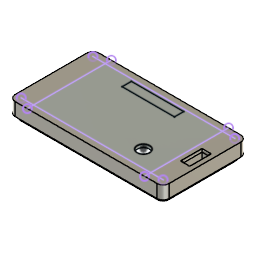
Flashlight (Autodesk Fusion 360 design; units mm, degrees)
Autodesk Fusion 360 part; units mm, degrees
note: some values were not read from the file. Set by a fixed rule: which sketch regions a step uses.
sketch "Sketch1" plane through (0, 0, 0) normal (0, 0, 1) x (1, 0, 0) in component "Bottom"
  line L0 (0, 0) -> (38.1, 0)
  line L1 (38.1, 0) -> (38.1, 27.3)
  line L2 (38.1, 27.3) -> (0, 27.3)
  line L3 (0, 27.3) -> (0, 0)
  line L4 (0, 0) -> (-4, 0)
  line L5 (-6, 2) -> (-6, 25.3)
  line L6 (-4, 27.3) -> (0, 27.3)
  line L7 (0, 27.3) -> (0, 0)
  line L8 (38.1, 0) -> (42.1, 0)
  line L9 (44.1, 2) -> (44.1, 25.3)
  line L10 (42.1, 27.3) -> (38.1, 27.3)
  line L11 (38.1, 27.3) -> (38.1, 0)
  line L12 (-4, 2) -> (42.1, 2)
  line L13 (42.1, 2) -> (42.1, 25.3)
  line L14 (42.1, 25.3) -> (-4, 25.3)
  line L15 (-4, 25.3) -> (-4, 2)
  line L16 (-4, 2) -> (0, 2)
  line L17 (0, 2) -> (0, 5)
  line L18 (-1, 6) -> (-4, 6)
  line L19 (-4, 6) -> (-4, 2)
  line L20 (-4, 25.3) -> (0, 25.3)
  line L21 (0, 25.3) -> (0, 22.3)
  line L22 (-1, 21.3) -> (-4, 21.3)
  line L23 (-4, 21.3) -> (-4, 25.3)
  line L24 (42.1, 25.3) -> (38.1, 25.3)
  line L25 (38.1, 25.3) -> (38.1, 22.3)
  line L26 (39.1, 21.3) -> (42.1, 21.3)
  line L27 (42.1, 21.3) -> (42.1, 25.3)
  line L28 (42.1, 2) -> (38.1, 2)
  line L29 (38.1, 2) -> (38.1, 5)
  line L30 (39.1, 6) -> (42.1, 6)
  line L31 (42.1, 6) -> (42.1, 2)
  arc A0 (-1, 21.3) -> (0, 22.3) centre (-1, 22.3) ccw
  arc A1 (38.1, 22.3) -> (39.1, 21.3) centre (39.1, 22.3) ccw
  arc A2 (39.1, 6) -> (38.1, 5) centre (39.1, 5) ccw
  arc A3 (0, 5) -> (-1, 6) centre (-1, 5) ccw
  arc A4 (-4, 27.3) -> (-6, 25.3) centre (-4, 25.3) ccw
  arc A5 (44.1, 25.3) -> (42.1, 27.3) centre (42.1, 25.3) ccw
  arc A6 (42.1, 0) -> (44.1, 2) centre (42.1, 2) ccw
  arc A7 (-6, 2) -> (-4, 0) centre (-4, 2) ccw
  line L32 (-3.5, 26.55) -> (41.6, 26.55)
  line L33 (43.35, 24.8) -> (43.35, 2.5)
  line L34 (41.6, 0.75) -> (-3.5, 0.75)
  line L35 (-5.25, 2.5) -> (-5.25, 24.8)
  arc A8 (-3.5, 26.55) -> (-5.25, 24.8) centre (-3.5, 24.8) ccw
  arc A9 (43.35, 24.8) -> (41.6, 26.55) centre (41.6, 24.8) ccw
  arc A10 (41.6, 0.75) -> (43.35, 2.5) centre (41.6, 2.5) ccw
  arc A11 (-5.25, 2.5) -> (-3.5, 0.75) centre (-3.5, 2.5) ccw
  line L36 (-1, 19) -> (22, 19)
  line L37 (22, 19) -> (22, 6.5)
  line L38 (22, 6.5) -> (-1, 6.5)
  line L39 (-1, 6.5) -> (-1, 19)
  line L40 (-1, 19) -> (22, 19)
  line L41 (22, 19) -> (22, 19.5)
  line L42 (22, 19.5) -> (-1, 19.5)
  line L43 (-1, 19.5) -> (-1, 19)
  line L44 (-1, 6.5) -> (22, 6.5)
  line L45 (22, 6.5) -> (22, 6)
  line L46 (22, 6) -> (-1, 6)
  line L47 (-1, 6) -> (-1, 6.5)
  line L48 (22, 19) -> (21.5, 19)
  line L49 (21.5, 19) -> (21.5, 6.5)
  line L50 (21.5, 6.5) -> (22, 6.5)
  line L51 (22, 6.5) -> (22, 19)
  line L52 (38.1, 25.3) -> (28.1, 25.3)
  line L53 (28.1, 25.3) -> (28.1, 23.3)
  line L54 (28.1, 23.3) -> (38.1, 23.3)
  line L55 (38.1, 23.3) -> (38.1, 25.3)
  line L56 (38.1, 2) -> (28.1, 2)
  line L57 (28.1, 2) -> (28.1, 4)
  line L58 (28.1, 4) -> (38.1, 4)
  line L59 (38.1, 4) -> (38.1, 2)
  line L60 (42.1, 18.65) -> (38.1, 18.65)
  line L61 (38.1, 18.65) -> (38.1, 8.65)
  line L62 (38.1, 8.65) -> (42.1, 8.65)
  line L63 (42.1, 8.65) -> (42.1, 18.65)
  line L64 (42.1, 16.65) -> (40.1, 16.65)
  line L65 (40.1, 16.65) -> (40.1, 10.65)
  line L66 (40.1, 10.65) -> (42.1, 10.65)
  line L67 (42.1, 10.65) -> (42.1, 16.65)
  point P0 (-6, 0)
  point P1 (-6, 27.3)
  point P2 (44.1, 0)
  point P3 (44.1, 27.3)
  point P4 (-5.25, 26.55)
  point P5 (43.35, 26.55)
  point P6 (-5.25, 0.75)
  dimension "d1" = 38.1
  dimension "d2" = 27.3
  dimension "d3" = 6
  dimension "d4" = 27.3
  dimension "d5" = 6
  dimension "d6" = 27.3
  dimension "d8" = 46.1
  dimension "d9" = 23.3
  dimension "d10" = 50.1
  dimension "d11" = 2
  dimension "d12" = 2
  dimension "d13" = 4
  dimension "d14" = 4
  dimension "d15" = 4
  dimension "d16" = 4
  dimension "d17" = 4
  dimension "d18" = 4
  dimension "d19" = 4
  dimension "d20" = 4
  dimension "d21" = 1
  dimension "d22" = 1
  dimension "d23" = 1
  dimension "d24" = 1
  dimension "d25" = 2
  dimension "d26" = 2
  dimension "d27" = 2
  dimension "d28" = 2
  dimension "d29" = 48.6
  dimension "d30" = 25.8
  dimension "d31" = 0.75
  dimension "d32" = 0.75
  dimension "d33" = 1.75
  dimension "d34" = 1.75
  dimension "d35" = 1.75
  dimension "d36" = 1.75
  dimension "d37" = 23
  dimension "d38" = 12.5
  dimension "d39" = 4.5
  dimension "d40" = 3
  dimension "d41" = 23
  dimension "d42" = 0.5
  dimension "d43" = 23
  dimension "d44" = 0.5
  dimension "d45" = 0.5
  dimension "d46" = 12.5
  dimension "d47" = 10
  dimension "d48" = 2
  dimension "d49" = 10
  dimension "d50" = 2
  dimension "d90" = 15.3
  dimension "d91" = 4
  dimension "d92" = 10
  dimension "d93" = 2.65
  dimension "d94" = 2
  dimension "d95" = 6
  dimension "d96" = 2
  constraint horizontal L0
  constraint vertical L1
  constraint horizontal L2
  constraint vertical L3
  constraint coincident L0.start L3.end
  constraint horizontal L4
  constraint vertical L5
  constraint horizontal L6
  constraint vertical L7
  constraint horizontal L8
  constraint vertical L9
  constraint horizontal L10
  constraint vertical L11
  constraint horizontal L12
  constraint vertical L13
  constraint horizontal L14
  constraint vertical L15
  constraint horizontal L16
  constraint vertical L17
  constraint horizontal L18
  constraint vertical L19
  constraint horizontal L20
  constraint vertical L21
  constraint horizontal L22
  constraint vertical L23
  constraint horizontal L24
  constraint vertical L25
  constraint horizontal L26
  constraint vertical L27
  constraint horizontal L28
  constraint vertical L29
  constraint horizontal L30
  constraint vertical L31
  constraint tangent L21 A0
  constraint tangent L22 A0
  constraint tangent L25 A1
  constraint tangent L26 A1
  constraint tangent L29 A2
  constraint tangent L30 A2
  constraint tangent L17 A3
  constraint tangent L18 A3
  constraint coincident P1 L5
  constraint coincident P1 L6
  constraint tangent L5 A4
  constraint tangent L6 A4
  constraint coincident P3 L9
  constraint coincident P3 L10
  constraint tangent L9 A5
  constraint tangent L10 A5
  constraint coincident P2 L8
  constraint coincident P2 L9
  constraint tangent L8 A6
  constraint tangent L9 A6
  constraint coincident P0 L4
  constraint coincident P0 L5
  constraint tangent L4 A7
  constraint tangent L5 A7
  constraint horizontal L32
  constraint vertical L33
  constraint horizontal L34
  constraint vertical L35
  constraint coincident P4 L32
  constraint coincident P4 L35
  constraint tangent L32 A8
  constraint tangent L35 A8
  constraint coincident P5 L32
  constraint coincident P5 L33
  constraint tangent L32 A9
  constraint tangent L33 A9
  constraint tangent L33 A10
  constraint tangent L34 A10
  constraint coincident P6 L34
  constraint coincident P6 L35
  constraint tangent L34 A11
  constraint tangent L35 A11
  constraint horizontal L36
  constraint vertical L37
  constraint horizontal L38
  constraint vertical L39
  constraint horizontal L40
  constraint vertical L41
  constraint horizontal L42
  constraint vertical L43
  constraint horizontal L44
  constraint vertical L45
  constraint horizontal L46
  constraint vertical L47
  constraint horizontal L48
  constraint vertical L49
  constraint horizontal L50
  constraint vertical L51
  constraint horizontal L52
  constraint vertical L53
  constraint horizontal L54
  constraint vertical L55
  constraint horizontal L56
  constraint vertical L57
  constraint horizontal L58
  constraint vertical L59
  constraint horizontal L60
  constraint vertical L61
  constraint horizontal L62
  constraint vertical L63
  constraint coincident L13 L60.start
  constraint horizontal L64
  constraint vertical L65
  constraint horizontal L66
  constraint vertical L67
  constraint coincident L63 L64.start
  measures "d1" distance of L0.start L0.end
  measures "d2" distance of L0.start L2.end
  measures "d3" distance of L0.start P0
  measures "d4" distance of L0.start L2.end
  measures "d5" distance of L0.end P2
  measures "d6" distance of L0.end L1.end
  measures "d8" distance of L12.start L12.end
  measures "d9" distance of L12.start L14.end
  measures "d10" distance of P1 P3
  measures "d11" distance of L4 L12
  measures "d12" distance of L5 L15
  measures "d13" distance of L12.start L16.end
  measures "d14" distance of L12.start L18.end
  measures "d15" distance of L14.end L20.end
  measures "d16" distance of L14.end L22.end
  measures "d17" distance of L13.end L24.end
  measures "d18" distance of L13.end L26.end
  measures "d19" distance of L12.end L28.end
  measures "d20" distance of L12.end L30.end
  measures "d21" radius of A0
  measures "d22" radius of A1
  measures "d23" radius of A2
  measures "d24" radius of A3
  measures "d25" radius of A4
  measures "d26" radius of A5
  measures "d27" radius of A6
  measures "d28" radius of A7
  measures "d29" distance of P4 P5
  measures "d30" distance of P4 P6
  measures "d31" distance of L2 L32
  measures "d32" distance of L5 L35
  measures "d33" radius of A8
  measures "d34" radius of A9
  measures "d35" radius of A10
  measures "d36" radius of A11
  measures "d37" distance of L36.start L36.end
  measures "d38" distance of L36.start L38.end
  measures "d39" distance of L12 L38
  measures "d40" distance of L15 L39
  measures "d41" distance of L36.start L36.end
  measures "d42" distance of L36.start L42.end
  measures "d43" distance of L38.end L37.end
  measures "d44" distance of L38.end L18.start
  measures "d45" distance of L36.end L48.end
  measures "d46" distance of L36.end L37.end
  measures "d47" distance of L24.end L52.end
  measures "d48" distance of L24.end L54.end
  measures "d49" distance of L28.end L56.end
  measures "d50" distance of L28.end L58.end
  measures "d90" distance of L26 L30
  measures "d91" distance of L60.start L60.end
  measures "d92" distance of L60.start L62.end
  measures "d93" distance of L26 L60
  measures "d94" distance of L64.start L64.end
  measures "d95" distance of L64.start L66.end
  measures "d96" distance of L60 L64
extrude "Extrude1" add sketch "Sketch1" against normal blind 1 makes body 1 in component "Bottom"
extrude "Extrude2" add sketch "Sketch1" along normal blind 5.5 contours L3 L7 L38 L44 L46 L47 | L3 L7 L38 L44 L45 L46 L50 | L3 L7 L36 L40 L42 L43 | L3 L7 L36 L40 L41 L42 L48 | L36 L37 L38 L40 L44 L48 L49 L50 L51 bodies 1 in component "Bottom"
extrude "Extrude3" add sketch "Sketch1" along normal blind 5.5 contours L1 L11 L12 L29 L56 L57 L58 L59 | L1 L11 L14 L25 L52 L53 L54 L55 bodies 1 in component "Bottom"
extrude "Extrude4" add sketch "Sketch1" along normal blind 7.1 separate body contours L3 L7 L12 L14 L15 L16 L19 L20 L23 L32 L34 L35 A8 A11 | L1 L3 L7 L11 L12 L34 L56 | L1 L11 L12 L13 L14 L24 L27 L28 L31 L32 L33 L34 A9 A10 L63 L67 | L3 L7 L12 L15 L16 L17 L18 L19 A3 | L1 L11 L12 L13 L28 L29 L30 L31 A2 L59 | L3 L7 L14 L15 L20 L21 L22 L23 A0 | L1 L3 L7 L11 L14 L32 L52 | L1 L11 L13 L14 L24 L25 L26 L27 A1 L55 makes body 2 in component "Bottom"
extrude "Extrude5" add sketch "Sketch1" along normal blind 8.1 contours L0 L1 L3 L7 L11 L34 | L3 L4 L5 L6 L7 A4 A7 L32 L34 L35 A8 A11 | L1 L8 L9 L10 L11 A5 A6 L32 L33 L34 A9 A10 | L1 L2 L3 L7 L11 L32 bodies 1 2 in component "Bottom"
sketch "Sketch2" plane through (0, 0, 8.1) normal (0, 0, 1) x (-1, 0, 0) in component "Bottom"
  arc A0 (3.5, -26.55) -> (5.25, -24.8) centre (3.5, -24.8) ccw
  line L0 (3.5, -26.55) -> (-41.6, -26.55)
  arc A1 (-43.35, -24.8) -> (-41.6, -26.55) centre (-41.6, -24.8) ccw
  line L1 (-43.35, -24.8) -> (-43.35, -2.5)
  arc A2 (-41.6, -0.75) -> (-43.35, -2.5) centre (-41.6, -2.5) ccw
  line L2 (-41.6, -0.75) -> (3.5, -0.75)
  arc A3 (5.25, -2.5) -> (3.5, -0.75) centre (3.5, -2.5) ccw
  line L3 (5.25, -2.5) -> (5.25, -24.8)
  arc A4 (4, -27.3) -> (6, -25.3) centre (4, -25.3) ccw
  line L4 (6, -25.3) -> (6, -2)
  arc A5 (6, -2) -> (4, 0) centre (4, -2) ccw
  line L5 (4, 0) -> (-42.1, 0)
  arc A6 (-42.1, 0) -> (-44.1, -2) centre (-42.1, -2) ccw
  line L6 (-44.1, -2) -> (-44.1, -25.3)
  arc A7 (-44.1, -25.3) -> (-42.1, -27.3) centre (-42.1, -25.3) ccw
  line L7 (-42.1, -27.3) -> (4, -27.3)
  line L8 (-1, -27.3) -> (-9.2, -27.3)
  line L9 (-9.2, -27.3) -> (-9.2, -25.3)
  line L10 (-9.2, -25.3) -> (-1, -25.3)
  line L11 (-1, -25.3) -> (-1, -27.3)
  line L12 (0, -27.3) -> (0, 0)
  dimension "d61" = 8.2
  dimension "d62" = 2
  dimension "d63" = 1
  constraint horizontal L8
  constraint vertical L9
  constraint horizontal L10
  constraint vertical L11
  constraint coincident L7 L8.start
  measures "d61" distance of L8.start L8.end
  measures "d62" distance of L8.start L10.end
  measures "d63" distance of L11 L12
extrude "Extrude6" cut sketch "Sketch2" against normal blind 1.2 contours L0 L7 L8 L9 L11 | L0 L9 L10 L11 bodies 1 in component "Bottom"
sketch "Sketch3" plane through (0, 0, -1) normal (0, 0, -1) x (1, 0, 0) in component "Bottom"
  arc A0 (-6, -25.3) -> (-4, -27.3) centre (-4, -25.3) ccw
  line L0 (-4, -27.3) -> (42.1, -27.3)
  arc A1 (42.1, -27.3) -> (44.1, -25.3) centre (42.1, -25.3) ccw
  line L1 (44.1, -25.3) -> (44.1, -2)
  arc A2 (44.1, -2) -> (42.1, 0) centre (42.1, -2) ccw
  line L2 (42.1, 0) -> (-4, 0)
  arc A3 (-4, 0) -> (-6, -2) centre (-4, -2) ccw
  line L3 (-6, -2) -> (-6, -25.3)
  circle A4 centre (-3, -3) radius 2.5
  line L4 (0, 0) -> (-4, 0)
  line L5 (-6, -2) -> (-6, -25.3)
  circle A5 centre (-3, -3) radius 1
  circle A6 centre (41.1, -3) radius 2.5
  line L6 (38.1, 0) -> (42.1, 0)
  line L7 (44.1, -2) -> (44.1, -25.3)
  circle A7 centre (41.1, -3) radius 1
  circle A8 centre (41.1, -24.3) radius 2.5
  line L8 (42.1, -27.3) -> (38.1, -27.3)
  circle A9 centre (41.1, -24.3) radius 1
  circle A10 centre (-3, -24.3) radius 2.5
  line L9 (-4, -27.3) -> (0, -27.3)
  circle A11 centre (-3, -24.3) radius 1
  dimension "d66" = 5
  dimension "d67" = 3
  dimension "d68" = 3
  dimension "d69" = 2
  dimension "d70" = 5
  dimension "d71" = 3
  dimension "d72" = 3
  dimension "d73" = 2
  dimension "d74" = 5
  dimension "d75" = 3
  dimension "d76" = 3
  dimension "d77" = 2
  dimension "d78" = 5
  dimension "d79" = 3
  dimension "d80" = 3
  dimension "d81" = 2
  constraint concentric A4 A5
  constraint concentric A6 A7
  constraint concentric A8 A9
  constraint concentric A10 A11
  measures "d66" diameter of A4
  measures "d67" distance of A4.centre L4
  measures "d68" distance of A4.centre L5
  measures "d69" diameter of A5
  measures "d70" diameter of A6
  measures "d71" distance of A6.centre L6
  measures "d72" distance of A6.centre L7
  measures "d73" diameter of A7
  measures "d74" diameter of A8
  measures "d75" distance of L7 A8.centre
  measures "d76" distance of A8.centre L8
  measures "d77" diameter of A9
  measures "d78" diameter of A10
  measures "d79" distance of L5 A10.centre
  measures "d80" distance of A10.centre L9
  measures "d81" diameter of A11
extrude "Extrude7" cut sketch "Sketch3" against normal blind 9.5 contours A5 | A7 | A9 | A11 bodies 1 in component "Bottom"
extrude "Extrude8" cut sketch "Sketch3" against normal blind 5 contours A4 | A6 | A8 | A10 bodies 1 in component "Bottom"
chamfer "Chamfer1" distance 1.5 angle 45 1 edges at (-3.9323, 24.6616, 4) on bodies 1 in component "Bottom"
chamfer "Chamfer2" distance 1.5 angle 45 1 edges at (-3.9323, 3.3616, 4) on bodies 1 in component "Bottom"
chamfer "Chamfer3" distance 1.5 angle 45 1 edges at (40.1677, 24.6616, 4) on bodies 1 in component "Bottom"
chamfer "Chamfer4" distance 1.5 angle 45 1 edges at (40.1677, 3.3616, 4) on bodies 1 in component "Bottom"
extrude "Extrude9" cut sketch "Sketch1" against normal blind 1 contours L13 L63 L64 L65 L66 L67 bodies 1 in component "Bottom"
extrude "Extrude10" add sketch "Sketch1" along normal blind 7.1 separate body contours L1 L11 L13 L60 L61 L62 L63 L64 L65 L66 makes body 3 in component "Bottom"
fillet "Fillet1" radius 0.5 4 edges at (40.1, 13.65, -1) (41.1, 16.65, -1) (42.1, 13.65, -1) (41.1, 10.65, -1) on bodies 1 in component "Bottom"
sketch "Sketch1 (2)" plane through (0, 0, 0) normal (0, 0, 1) x (1, 0, 0) in component "Top"
  line L0 (-4, 6) -> (19, 6)
  arc A0 (-7, 26.8) -> (-9, 24.8) centre (-7, 24.8) ccw
  line L1 (39.1, 20.8) -> (39.1, 24.8)
  line L2 (39.1, 16.15) -> (37.1, 16.15)
  line L3 (39.1, 26.8) -> (35.1, 26.8)
  arc A1 (-6.25, 25.8) -> (-8, 24.05) centre (-6.25, 24.05) ccw
  line L4 (19, 6) -> (19, 5.5)
  line L5 (19, 18.5) -> (19, 6)
  line L6 (-7, 26.8) -> (-3, 26.8)
  arc A2 (-4, 20.8) -> (-3, 21.8) centre (-4, 21.8) ccw
  line L7 (39.1, 24.8) -> (-7, 24.8)
  line L8 (-9, 1.5) -> (-9, 24.8)
  line L9 (-3, 26.8) -> (-3, -0.5)
  arc A3 (38.35, 0.5) -> (40.1, 2.25) centre (38.35, 2.25) ccw
  line L10 (39.1, 8.15) -> (39.1, 18.15)
  line L11 (-4, 6) -> (-4, 18.5)
  line L12 (-4, 19) -> (-4, 18.5)
  line L13 (19, 6) -> (-4, 6)
  line L14 (33.1, 6.5) -> (35.1, 6.5)
  line L15 (-4, 5.5) -> (-4, 6)
  line L16 (40.1, 24.05) -> (40.1, 2.25)
  line L17 (-7, 1.5) -> (39.1, 1.5)
  line L18 (36.1, 20.8) -> (39.1, 20.8)
  line L19 (19, 6) -> (19, 18.5)
  line L20 (-4, 18.5) -> (19, 18.5)
  line L21 (-4, 18.5) -> (19, 18.5)
  line L22 (-8, 2.25) -> (-8, 24.05)
  line L23 (38.35, 0.5) -> (-6.25, 0.5)
  line L24 (35.1, -0.5) -> (35.1, 26.8)
  line L25 (35.1, -0.5) -> (39.1, -0.5)
  line L26 (-3, -0.5) -> (-7, -0.5)
  line L27 (39.1, 5.5) -> (39.1, 1.5)
  line L28 (35.1, 26.8) -> (-3, 26.8)
  line L29 (-3, 1.5) -> (-3, 4.5)
  line L30 (-3, -0.5) -> (35.1, -0.5)
  arc A4 (40.1, 24.05) -> (38.35, 25.8) centre (38.35, 24.05) ccw
  line L31 (-7, 5.5) -> (-7, 1.5)
  line L32 (-3, 26.8) -> (-3, -0.5)
  arc A5 (-8, 2.25) -> (-6.25, 0.5) centre (-6.25, 2.25) ccw
  line L33 (-7, 24.8) -> (-7, 1.5)
  line L34 (39.1, 1.5) -> (35.1, 1.5)
  line L35 (41.1, 1.5) -> (41.1, 24.8)
  arc A6 (39.1, -0.5) -> (41.1, 1.5) centre (39.1, 1.5) ccw
  line L36 (35.1, 18.15) -> (35.1, 8.15)
  line L37 (37.1, 16.15) -> (37.1, 10.15)
  line L38 (35.1, 24.8) -> (35.1, 21.8)
  arc A7 (36.1, 5.5) -> (35.1, 4.5) centre (36.1, 4.5) ccw
  line L39 (-7, 1.5) -> (-3, 1.5)
  line L40 (-4, 20.8) -> (-7, 20.8)
  line L41 (36.1, 5.5) -> (39.1, 5.5)
  line L42 (-7, 24.8) -> (-3, 24.8)
  line L43 (35.1, 26.8) -> (35.1, -0.5)
  line L44 (39.1, 10.15) -> (39.1, 16.15)
  line L45 (28.1, 24.8) -> (28.1, 22.8)
  line L46 (35.1, 22.8) -> (35.1, 24.8)
  arc A8 (-9, 1.5) -> (-7, -0.5) centre (-7, 1.5) ccw
  line L47 (-7, 20.8) -> (-7, 24.8)
  line L48 (19, 18.5) -> (18.5, 18.5)
  line L49 (19, 5.5) -> (-4, 5.5)
  line L50 (18.5, 6) -> (19, 6)
  line L51 (33.1, 1.5) -> (33.1, 6.5)
  line L52 (35.1, 1.5) -> (35.1, 4.5)
  line L53 (18.5, 18.5) -> (18.5, 6)
  arc A9 (-3, 4.5) -> (-4, 5.5) centre (-4, 4.5) ccw
  line L54 (-6.25, 25.8) -> (38.35, 25.8)
  line L55 (35.1, 8.15) -> (39.1, 8.15)
  line L56 (35.1, 24.8) -> (28.1, 24.8)
  line L57 (-4, 5.5) -> (-7, 5.5)
  line L58 (35.1, 1.5) -> (33.1, 1.5)
  arc A10 (41.1, 24.8) -> (39.1, 26.8) centre (39.1, 24.8) ccw
  line L59 (19, 18.5) -> (19, 19)
  line L60 (-3, 24.8) -> (-3, 21.8)
  line L61 (35.1, 6.5) -> (35.1, 1.5)
  line L62 (39.1, 24.8) -> (35.1, 24.8)
  line L63 (37.1, 10.15) -> (39.1, 10.15)
  line L64 (39.1, 1.5) -> (39.1, 24.8)
  line L65 (28.1, 22.8) -> (35.1, 22.8)
  line L66 (19, 19) -> (-4, 19)
  line L67 (39.1, 18.15) -> (35.1, 18.15)
  arc A11 (35.1, 21.8) -> (36.1, 20.8) centre (36.1, 21.8) ccw
  line L68 (7, 9) -> (9, 9)
  line L69 (9, 9) -> (9, 11)
  line L70 (9, 11) -> (7, 11)
  line L71 (7, 11) -> (7, 9)
  point P0 (41.1, 26.8)
  point P1 (41.1, -0.5)
  point P2 (-3, -0.5)
  point P3 (-8, 0.5)
  point P4 (-8, 25.8)
  point P5 (40.1, 25.8)
  point P6 (-9, -0.5)
  point P7 (-9, 26.8)
  dimension "d103" = 38.1
  dimension "d104" = 27.3
  dimension "d105" = 6
  dimension "d106" = 27.3
  dimension "d107" = 6
  dimension "d108" = 27.3
  dimension "d109" = 46.1
  dimension "d110" = 23.3
  dimension "d111" = 50.1
  dimension "d112" = 2
  dimension "d113" = 2
  dimension "d114" = 4
  dimension "d115" = 4
  dimension "d116" = 4
  dimension "d117" = 4
  dimension "d118" = 4
  dimension "d119" = 4
  dimension "d120" = 4
  dimension "d121" = 4
  dimension "d122" = 1
  dimension "d123" = 1
  dimension "d124" = 1
  dimension "d125" = 1
  dimension "d126" = 2
  dimension "d127" = 2
  dimension "d128" = 2
  dimension "d129" = 2
  dimension "d130" = 48.1
  dimension "d131" = 25.3
  dimension "d132" = 1
  dimension "d133" = 1
  dimension "d134" = 1.75
  dimension "d135" = 1.75
  dimension "d136" = 1.75
  dimension "d137" = 1.75
  dimension "d138" = 23
  dimension "d139" = 12.5
  dimension "d140" = 4.5
  dimension "d141" = 3
  dimension "d142" = 23
  dimension "d143" = 0.5
  dimension "d144" = 23
  dimension "d145" = 0.5
  dimension "d146" = 0.5
  dimension "d147" = 12.5
  dimension "d148" = 7
  dimension "d149" = 2
  dimension "d150" = 2
  dimension "d151" = 5
  dimension "d152" = 15.3
  dimension "d153" = 4
  dimension "d154" = 10
  dimension "d155" = 2.65
  dimension "d156" = 2
  dimension "d157" = 6
  dimension "d158" = 2
  dimension "d188" = 2
  dimension "d189" = 2
  dimension "d190" = 10
  dimension "d191" = 7.5
  constraint horizontal L30
  constraint vertical L24
  constraint horizontal L28
  constraint vertical L9
  constraint coincident P2 L9.end
  constraint horizontal L26
  constraint vertical L8
  constraint horizontal L6
  constraint vertical L32
  constraint horizontal L25
  constraint vertical L35
  constraint horizontal L3
  constraint vertical L43
  constraint horizontal L17
  constraint vertical L64
  constraint horizontal L7
  constraint vertical L33
  constraint horizontal L39
  constraint vertical L29
  constraint horizontal L57
  constraint vertical L31
  constraint horizontal L42
  constraint vertical L60
  constraint horizontal L40
  constraint vertical L47
  constraint horizontal L62
  constraint vertical L38
  constraint horizontal L18
  constraint vertical L1
  constraint horizontal L34
  constraint vertical L52
  constraint horizontal L41
  constraint vertical L27
  constraint tangent A2 L60
  constraint tangent A2 L40
  constraint tangent L38 A11
  constraint tangent L18 A11
  constraint tangent A7 L52
  constraint tangent A7 L41
  constraint tangent L29 A9
  constraint tangent A9 L57
  constraint coincident P7 L8
  constraint coincident P7 L6
  constraint tangent A0 L8
  constraint tangent A0 L6
  constraint coincident P0 L35
  constraint coincident P0 L3
  constraint tangent L35 A10
  constraint tangent L3 A10
  constraint coincident P1 L25
  constraint coincident P1 L35
  constraint tangent L25 A6
  constraint tangent L35 A6
  constraint coincident P6 L26
  constraint coincident P6 L8
  constraint tangent L26 A8
  constraint tangent L8 A8
  constraint horizontal L54
  constraint vertical L16
  constraint horizontal L23
  constraint vertical L22
  constraint coincident P4 L54
  constraint coincident P4 L22
  constraint tangent A1 L54
  constraint tangent A1 L22
  constraint coincident P5 L54
  constraint coincident P5 L16
  constraint tangent A4 L54
  constraint tangent L16 A4
  constraint tangent A3 L16
  constraint tangent A3 L23
  constraint coincident P3 L23
  constraint coincident P3 L22
  constraint tangent L23 A5
  constraint tangent L22 A5
  constraint horizontal L21
  constraint vertical L5
  constraint horizontal L13
  constraint vertical L11
  constraint horizontal L20
  constraint vertical L59
  constraint horizontal L66
  constraint vertical L12
  constraint horizontal L0
  constraint vertical L4
  constraint horizontal L49
  constraint vertical L15
  constraint horizontal L48
  constraint vertical L53
  constraint horizontal L50
  constraint vertical L19
  constraint horizontal L56
  constraint vertical L45
  constraint horizontal L65
  constraint vertical L46
  constraint horizontal L58
  constraint vertical L51
  constraint horizontal L14
  constraint vertical L61
  constraint horizontal L67
  constraint vertical L36
  constraint horizontal L55
  constraint vertical L10
  constraint coincident L10.end L64
  constraint horizontal L2
  constraint vertical L37
  constraint horizontal L63
  constraint vertical L44
  constraint coincident L2.start L10
  constraint horizontal L68
  constraint vertical L69
  constraint horizontal L70
  constraint vertical L71
  measures "d103" distance of L24.start P2
  measures "d104" distance of L6.end P2
  measures "d105" distance of P6 P2
  measures "d106" distance of L6.end P2
  measures "d107" distance of P1 L24.start
  measures "d108" distance of L3.end L24.start
  measures "d109" distance of L17.start L17.end
  measures "d110" distance of A0.centre L17.start
  measures "d111" distance of P0 P7
  measures "d112" distance of L17 L26
  measures "d113" distance of L8 L33
  measures "d114" distance of L29.start L17.start
  measures "d115" distance of L31.start L17.start
  measures "d116" distance of L42.end A0.centre
  measures "d117" distance of L40.end A0.centre
  measures "d118" distance of L38.start L1.end
  measures "d119" distance of L1.start L1.end
  measures "d120" distance of L34.end L17.end
  measures "d121" distance of L27.start L17.end
  measures "d122" radius of A2
  measures "d123" radius of A11
  measures "d124" radius of A7
  measures "d125" radius of A9
  measures "d126" radius of A0
  measures "d127" radius of A10
  measures "d128" radius of A6
  measures "d129" radius of A8
  measures "d130" distance of P4 P5
  measures "d131" distance of P3 P4
  measures "d132" distance of L28 L54
  measures "d133" distance of L8 L22
  measures "d134" radius of A1
  measures "d135" radius of A4
  measures "d136" radius of A3
  measures "d137" radius of A5
  measures "d138" distance of L5.start L11.end
  measures "d139" distance of L11.end L0.start
  measures "d140" distance of L13 L17
  measures "d141" distance of L11 L33
  measures "d142" distance of L5.start L11.end
  measures "d143" distance of L11.end L12.start
  measures "d144" distance of L0.end L0.start
  measures "d145" distance of L15.start L0.start
  measures "d146" distance of L5.start L48.end
  measures "d147" distance of L5.start L0.end
  measures "d148" distance of L45.start L38.start
  measures "d149" distance of L46.start L38.start
  measures "d150" distance of L34.end L51.start
  measures "d151" distance of L34.end L14.end
  measures "d152" distance of L18 L41
  measures "d153" distance of L36.start L10.end
  measures "d154" distance of L10.start L10.end
  measures "d155" distance of L18 L67
  measures "d156" distance of L2.start L2.end
  measures "d157" distance of L2.start L44.start
  measures "d158" distance of L2 L67
  measures "d188" distance of L68.start L68.end
  measures "d189" distance of L68.start L70.end
  measures "d190" distance of L32 L71
  measures "d191" distance of L17 L68
extrude "Extrude1'" add sketch "Sketch1 (2)" against normal blind 1 separate body contours L0 L5 L13 L19 L20 L21 L48 L50 L53 | L0 L4 L9 L13 L32 L49 L50 | L0 L9 L13 L20 L21 L32 L53 | L4 L5 L7 L9 L14 L17 L19 L24 L29 L32 L36 L38 L43 L45 L49 L51 L59 L60 L65 L66 | L0 L9 L13 L15 L32 L49 | L0 L9 L11 L13 L20 L21 L32 | L9 L20 L21 L32 L48 L59 L66 | A2 L9 L11 L12 L15 L32 L33 L40 L57 L66 | L9 L12 L20 L21 L32 L66 | L9 L32 L49 A9 | L9 L17 L29 L31 L32 L33 L39 A9 L57 | A1 L7 L9 L17 L22 L23 L31 L32 A5 L33 L39 L42 L47 L54 | A2 L7 L9 L32 L33 L40 L42 L47 L60 | L9 L17 L23 L24 L32 L43 L58 | L7 L9 L24 L32 L43 L54 L56 | L9 L23 L24 L30 L32 L43 | A0 A1 L6 L8 L9 L22 L23 L26 L32 A5 A8 L54 | L14 L17 L24 L43 L51 L52 L58 L61 | L7 L24 L38 L43 L45 L46 L56 L65 | L9 L24 L28 L32 L43 L54 | L1 L7 A3 L10 L16 L17 L23 L24 L27 A4 L34 L43 L44 L54 L62 L64 | L3 A3 L16 L23 L24 L25 A4 L35 A6 L43 L54 A10 | L17 L24 L27 L34 A7 L41 L43 L52 L61 L64 | L1 L7 L18 L24 L38 L43 L46 L62 L64 A11 | L24 A7 L41 L43 L55 L61 L64 | L2 L10 L24 L36 L37 L43 L55 L63 L64 L67 | L18 L24 L43 L64 L67 A11 | L2 L10 L37 L44 L63 L64 | L68 L69 L70 L71 makes body 4 in component "Top"
extrude "Extrude2'" add sketch "Sketch1 (2)" against normal blind 5.5 contours L9 L17 L29 L31 L32 L33 L39 A9 L57 | A1 L7 L9 L17 L22 L23 L31 L32 A5 L33 L39 L42 L47 L54 | A2 L7 L9 L32 L33 L40 L42 L47 L60 | L9 L17 L23 L24 L32 L43 L58 | L7 L9 L24 L32 L43 L54 L56 | L1 L7 A3 L10 L16 L17 L23 L24 L27 A4 L34 L43 L44 L54 L62 L64 | L17 L24 L27 L34 A7 L41 L43 L52 L61 L64 | L1 L7 L18 L24 L38 L43 L46 L62 L64 A11 | L2 L10 L24 L36 L37 L43 L55 L63 L64 L67 bodies 4 in component "Top"
extrude "Extrude3'" cut sketch "Sketch1 (2)" against normal blind 1 contours L2 L10 L37 L44 L63 L64 bodies 4 in component "Top"
extrude "Extrude4'" add 1 faces at (8.6167, -0.1667, -1) along direction (0, 0, -1) blind 3.25 on bodies 4 bodies 4 in component "Top"
sketch "Sketch2 (2)" plane through (0, 0, -5.5) normal (0, 0, -1) x (1, 0, 0) in component "Top"
  line L0 (37.1, -10.15) -> (39.1, -10.15)
  line L1 (39.1, -10.15) -> (39.1, -16.15)
  line L2 (39.1, -16.15) -> (37.1, -16.15)
  line L3 (37.1, -16.15) -> (37.1, -10.15)
  line L4 (35.1, -21.8) -> (35.1, -24.8)
  line L5 (35.1, -24.8) -> (-3, -24.8)
  line L6 (-3, -24.8) -> (-3, -21.8)
  arc A0 (-3, -21.8) -> (-4, -20.8) centre (-4, -21.8) ccw
  line L7 (-4, -20.8) -> (-7, -20.8)
  line L8 (-7, -20.8) -> (-7, -5.5)
  line L9 (-7, -5.5) -> (-4, -5.5)
  arc A1 (-4, -5.5) -> (-3, -4.5) centre (-4, -4.5) ccw
  line L10 (-3, -4.5) -> (-3, -1.5)
  line L11 (-3, -1.5) -> (35.1, -1.5)
  line L12 (35.1, -1.5) -> (35.1, -4.5)
  arc A2 (35.1, -4.5) -> (36.1, -5.5) centre (36.1, -4.5) ccw
  line L13 (36.1, -5.5) -> (39.1, -5.5)
  line L14 (39.1, -5.5) -> (39.1, -8.15)
  line L15 (39.1, -8.15) -> (35.1, -8.15)
  line L16 (35.1, -8.15) -> (35.1, -18.15)
  line L17 (35.1, -18.15) -> (39.1, -18.15)
  line L18 (39.1, -18.15) -> (39.1, -20.8)
  line L19 (39.1, -20.8) -> (36.1, -20.8)
  arc A3 (36.1, -20.8) -> (35.1, -21.8) centre (36.1, -21.8) ccw
  arc A4 (-6.25, -0.5) -> (-8, -2.25) centre (-6.25, -2.25) ccw
  line L20 (-8, -2.25) -> (-8, -24.05)
  arc A5 (-8, -24.05) -> (-6.25, -25.8) centre (-6.25, -24.05) ccw
  line L21 (-6.25, -25.8) -> (38.35, -25.8)
  arc A6 (38.35, -25.8) -> (40.1, -24.05) centre (38.35, -24.05) ccw
  line L22 (40.1, -24.05) -> (40.1, -2.25)
  arc A7 (40.1, -2.25) -> (38.35, -0.5) centre (38.35, -2.25) ccw
  line L23 (38.35, -0.5) -> (-6.25, -0.5)
  circle A8 centre (-6, -2.5) radius 1
  line L24 (-9, -1.5) -> (-9, -24.8)
  line L25 (-3, 0.5) -> (-7, 0.5)
  circle A9 centre (38.1, -2.5) radius 1
  line L26 (35.1, 0.5) -> (39.1, 0.5)
  line L27 (41.1, -1.5) -> (41.1, -24.8)
  circle A10 centre (38.1, -23.8) radius 1
  line L28 (39.1, -26.8) -> (35.1, -26.8)
  circle A11 centre (-6, -23.8) radius 1
  line L29 (-7, -26.8) -> (-3, -26.8)
  line L30 (-2, -24.8) -> (6.2, -24.8)
  line L31 (6.2, -24.8) -> (6.2, -26.8)
  line L32 (6.2, -26.8) -> (-2, -26.8)
  line L33 (-2, -26.8) -> (-2, -24.8)
  line L34 (-3, -26.8) -> (-3, 0.5)
  dimension "d167" = 2
  dimension "d168" = 3
  dimension "d169" = 3
  dimension "d170" = 2
  dimension "d171" = 3
  dimension "d172" = 3
  dimension "d173" = 2
  dimension "d174" = 3
  dimension "d175" = 3
  dimension "d176" = 2
  dimension "d177" = 3
  dimension "d178" = 3
  dimension "d181" = 8.2
  dimension "d182" = 2
  dimension "d183" = 1
  constraint horizontal L30
  constraint vertical L31
  constraint horizontal L32
  constraint vertical L33
  constraint coincident L5 L30.start
  measures "d167" diameter of A8
  measures "d168" distance of A8.centre L24
  measures "d169" distance of A8.centre L25
  measures "d170" diameter of A9
  measures "d171" distance of A9.centre L26
  measures "d172" distance of A9.centre L27
  measures "d173" diameter of A10
  measures "d174" distance of L27 A10.centre
  measures "d175" distance of A10.centre L28
  measures "d176" diameter of A11
  measures "d177" distance of A11.centre L29
  measures "d178" distance of L24 A11.centre
  measures "d181" distance of L30.start L30.end
  measures "d182" distance of L30.start L32.end
  measures "d183" distance of L33 L34
extrude "Extrude5'" cut sketch "Sketch2 (2)" against normal blind 4 contours A8 | A9 | A10 | A11 bodies 4 in component "Top"
extrude "Extrude6'" cut sketch "Sketch2 (2)" against normal blind 1.8 contours L5 L21 L30 L31 L33 | L21 L31 L32 L33 bodies 4 in component "Top"
extrude "Extrude7'" add sketch "Sketch1 (2)" against normal blind 5.5 contours L14 L17 L24 L43 L51 L52 L58 L61 | L7 L24 L38 L43 L45 L46 L56 L65 bodies 4 in component "Top"
extrude "Extrude8'" add sketch "Sketch1 (2)" against normal blind 5.5 contours L68 L69 L70 L71 bodies 4 in component "Top"
sketch "Sketch3 (2)" plane through (0, 0, 0) normal (0, 0, 1) x (1, 0, 0) in component "Top"
  line L0 (6.25, 24.05) -> (23.25, 24.05)
  line L1 (23.25, 24.05) -> (23.25, 21.05)
  line L2 (23.25, 21.05) -> (6.25, 21.05)
  line L3 (6.25, 21.05) -> (6.25, 24.05)
  line L4 (-3, 26.8) -> (-3, -0.5)
  line L5 (39.1, 24.8) -> (-7, 24.8)
  circle A0 centre (27.25, 6.95) radius 2
  line L6 (35.1, 26.8) -> (35.1, -0.5)
  line L7 (-7, 1.5) -> (39.1, 1.5)
  dimension "d194" = 17
  dimension "d195" = 3
  dimension "d196" = 9.25
  dimension "d197" = 0.75
  dimension "d202" = 4
  dimension "d203" = 7.85
  dimension "d204" = 5.45
  constraint horizontal L0
  constraint vertical L1
  constraint horizontal L2
  constraint vertical L3
  measures "d194" distance of L0.start L0.end
  measures "d195" distance of L0.start L2.end
  measures "d196" distance of L3 L4
  measures "d197" distance of L0 L5
  measures "d202" diameter of A0
  measures "d203" distance of A0.centre L6
  measures "d204" distance of A0.centre L7
fillet "Fillet1'" radius 0.5 4 edges at (37.1, 13.15, 0) (38.1, 16.15, 0) (39.1, 13.15, 0) (38.1, 10.15, 0) on bodies 4 in component "Top"
extrude "Extrude9'" cut sketch "Sketch3 (2)" against normal blind 1 contours L0 L1 L2 L3 bodies 4 in component "Top"
extrude "Extrude10'" cut sketch "Sketch3 (2)" against normal blind 1 contours A0 bodies 4 in component "Top"
extrude "Extrude11" cut sketch "Sketch2 (2)" against normal blind 3 contours L5 L21 L30 L31 L33 | L21 L31 L32 L33 bodies 4 in component "Top"
extrude "Extrude12" add sketch "Sketch3 (2)" against normal blind 1 contours L0 L1 L2 L3 bodies 4 in component "Top"
component "Bottom" placed x (1, 0, 0) y (0, 1, 0) z (0, 0, 1) at (0, 0, 0)
component "Top" placed x (1, 0, 0) y (0, 1, 0) z (0, 0, 1) at (0, 0, 0)
